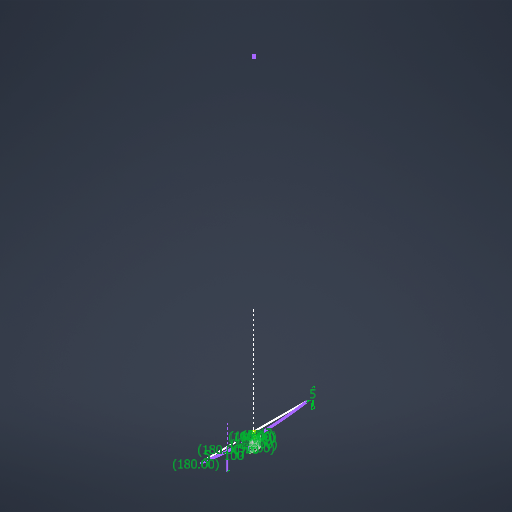
# Autodesk Inventor part: Pieza2
Saved by Autodesk Inventor 2026.1 (Build 301233020, 233B)
## iProperties
Created: 2026-05-16
Part Number: Pieza2
Material: Genérico
Document SubType Name: Modeling
Designer: USUARIO
Density: 1 g/cm^3
Appearance: Valor por defecto
Author: USUARIO
Autodesk Inventor part; units mm, degrees
ref_plane "YZ Plane" through (0, 0, 0) normal (1, 0, 0) x (0, 1, 0)
ref_plane "XZ Plane" through (0, 0, 0) normal (0, 1, 0) x (-1, 0, 0)
ref_plane "XY Plane" through (0, 0, 0) normal (0, 0, 1) x (1, 0, 0)
sketch "Boceto1" plane through (0, 0, 0) normal (1, 0, 0) x (0, 1, 0)
  line L0 (0, 0) -> (0, 125)
  line L1 (0, 0) -> (125, 0) construction
  line L2 (0, 0) -> (0, -125)
  line L3 (0, 0) -> (125, 0) construction
  line L4 (0, 0) -> (-20, 0)
  line L5 (0, 0) -> (20, 0) construction
  line L6 (0, 0) -> (500, 0) construction
  line L7 (0, 0) -> (-20, 0)
  line L8 (0, 0) -> (20, 0) construction
  line L9 (0, 0) -> (0, -246.4363)
  line L10 (0, 0) -> (246.4363, 0) construction
  line L11 (0, 0) -> (0, 250)
  line L12 (0, 0) -> (250, 0) construction
  arc A0 (0, 250) -> (0, -246.4363) centre (1530.2267, 1.7819) ccw
  line L13 (0, 125) -> (-100, 125)
  line L14 (0, 125) -> (100, 125) construction
  line L15 (0, 250) -> (-5, 250)
  line L16 (0, 250) -> (5, 250) construction
  line L17 (0, -246.4363) -> (-5, -246.4363)
  line L18 (-20, 0) -> (-23, 0)
  line L19 (-20, 0) -> (-17, 0) construction
  line L20 (-20, 0) -> (-25, 0)
  line L21 (-20, 0) -> (-15, 0) construction
  arc A1 (-5, 250) -> (-5, -246.4363) centre (1525.2267, 1.7819) ccw
  point P0 (-20.0963, 125)
  point P1 (-15.0963, 125)
  dimension "d14" = 100
  dimension "d15" = 180
  dimension "d16" = 5
  dimension "d17" = 180
  dimension "d18" = 5
  dimension "d19" = 3
  dimension "d20" = 180
  dimension "d21" = 5
  dimension "d22" = 180
  constraints: 44 end point, 17 horizontal, 10 equal length, 6 point on circle, 3 vertical, 2 centre point, 2 perpendicular
  measures "d14" distance of L0.end L13.end
  measures "d15" angle of L13 L14
  measures "d16" distance of L11.end L15.end
  measures "d17" angle of L15 L16
  measures "d18" distance of L9.end L17.end
  measures "d19" distance of L4.end L18.end
  measures "d20" angle of L18 L19
  measures "d21" distance of L4.end L20.end
  measures "d22" angle of L20 L21
revolve "Revolución1" add sketch "Boceto1" angle 90 about axis through (0, -20, 0) along (0, -1, 0) contours L18 L20 A1 L13 A0
fillet "Empalme1" [suppressed]
sketch "Boceto2" plane through (0, -25, 0) normal (1, 0, 0) x (0, 0, -1)
  line L0 (0, -0.001) -> (0, 4.7578) projected
  line L1 (0, -0.001) -> (25, -0.001) construction
  line L2 (0, -0.001) -> (0, -25.001)
  line L3 (0, -0.001) -> (25, -0.001) construction
  line L4 (-25, -50.001) -> (25, -50.001)
  line L5 (25, -50.001) -> (25, -0.001)
  line L6 (-25, -0.001) -> (-25, -50.001)
  line L7 (-25, -50.001) -> (25, -0.001) construction
  line L8 (25, -50.001) -> (-25, -0.001) construction
  arc A0 (-250.0001, 20) -> (246.437, 19.9995) centre (-1.7798, 1550.1723) ccw
  line L9 (-25, -0.001) -> (-25, 0.2817)
  line L10 (25, -0.001) -> (25, 0.5411)
  line L11 (0, -50.001) -> (0, -35.001)
  line L12 (0, -50.001) -> (15, -50.001) construction
  circle A1 centre (0, -35.001) radius 6
  line L13 (0, -35.001) -> (-20, -35.001)
  line L14 (0, -35.001) -> (20, -35.001) construction
  circle A2 centre (-20, -35.001) radius 2.5
  line L15 (-20.4375, -32.5396) -> (-1.05, -29.0936)
  line L16 (-20.4375, -37.4624) -> (0, -41.0951)
  line L17 (0, -35.001) -> (0, -29.001)
  line L18 (25, -50.001) -> (-25, -0.001) construction
  circle A3 centre (0, -35.001) radius 6
  line L19 (0, -35.001) -> (20, -35.001)
  circle A4 centre (20, -35.001) radius 2.5
  line L20 (20.4375, -32.5396) -> (1.05, -29.0936)
  line L21 (20.4375, -37.4624) -> (0, -41.0951)
  point P0 (0, 25)
  point P1 (0, 0)
  point P2 (-20.2213, -32.5012)
  point P3 (20.2213, -32.5012)
  point P4 (1.05, -29.0936)
  point P5 (25, 0.2293)
  point P6 (-25, 0.1719)
  point P7 (0, 4.9037)
  point P8 (-1.05, -40.9084)
  point P9 (1.05, -40.9084)
  dimension "d25" = 25
  dimension "d27" = 25
  dimension "d28" = 90
  dimension "d29" = 50
  dimension "d30" = 50
  dimension "d31" = 15
  dimension "d32" = 90
  dimension "d33" = 12
  dimension "d34" = 20
  dimension "d35" = 180
  dimension "d36" = 5
  constraints: 42 end point, 9 point on circle, 6 horizontal, 5 symmetric about line, 4 centre point, 4 point on line, 4 tangent, 3 coincident, 3 equal length, 3 midpoint, 3 vertical, 1 line through centre, 1 parallel, 1 perpendicular, 4 other
  measures "d25" distance of L0.start L2.end
  measures "d27" distance of L0.start L2.end
  measures "d28" angle of L2 L3
  measures "d29" distance of L6.start L3.end
  measures "d30" distance of L3.end L4.end
  measures "d31" distance of L11.start L11.end
  measures "d32" angle of L12 L11
  measures "d33" diameter of A1
  measures "d34" distance of L13.start L13.end
  measures "d35" angle of L13 L14
  measures "d36" diameter of A2
extrude "Extrusión1" add sketch "Boceto2" along normal blind 10
extrude "Extrusión2" add sketch "Boceto2" along normal blind 6 contours A1 L13 L11 | L11 L19 A1 | L16 A2 L13 A1 | A1 L19 A4 L21 | L13 A1 L17 | L17 A1 L19 | L13 A2 L15 A1 | A1 L20 A4 L19 | A4
sketch "Boceto3" plane through (0, -25, 0) normal (1, 0, 0) x (0, 0, -1)
  arc A0 (-25, 0.1719) -> (25, 0.2293) centre (-1.7798, 1550.1723) ccw projected
  line L0 (0, -0.001) -> (-143.598, -0.001)
  line L1 (-143.598, -0.001) -> (-143.598, 29.4802)
  line L2 (-143.598, 29.4802) -> (0, 29.4802)
  line L3 (0, 29.4802) -> (0, -0.001)
  point P0 (0, 25)
  constraints: 8 end point, 2 parallel, 1 horizontal, 1 perpendicular, 1 point on circle
extrude "Extrusión3" cut sketch "Boceto3" against normal blind 152
